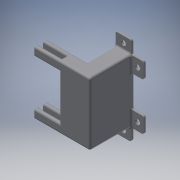
# Autodesk Inventor part: Tail_Base
Saved by Autodesk Inventor 2018 (Build 220112000, 112)
## iProperties
Created: 2017-11-24
Part Number: Tail_Base
Material: Generic
Document SubType Name: Modeling
Designer: reide
Density: 1 g/cm^3
Appearance: Default
Author: reide
Autodesk Inventor part; units mm, degrees
ref_plane "YZ Plane" through (0, 0, 0) normal (1, 0, 0) x (0, 1, 0)
ref_plane "XZ Plane" through (0, 0, 0) normal (0, 1, 0) x (-1, 0, 0)
ref_plane "XY Plane" through (0, 0, 0) normal (0, 0, 1) x (1, 0, 0)
sketch "Sketch1" plane through (0, 0, 0) normal (0, 0, 1) x (1, 0, 0)
  line L0 (0, -18.542) -> (0, -2.54) projected
  line L1 (0, -18.542) -> (-1.27, -18.542) projected
  line L2 (-11.43, -18.542) -> (-1.27, -18.542) projected
  line L3 (-11.43, -18.542) -> (-12.7, -18.542) projected
  line L4 (-12.7, -18.542) -> (-12.7, -2.54) projected
  line L5 (0, 0) -> (-12.7, 0) projected
  line L6 (-12.7, 0) -> (-12.7, -2.54) projected
  line L7 (0, -2.54) -> (-12.7, -2.54) projected
  line L8 (0, 0) -> (0, -2.54) projected
  line L9 (0, 0) -> (0, 4.318) projected
  line L10 (-6.35, 4.318) -> (-1.27, 4.318) projected
  line L11 (0, 4.318) -> (-1.27, 4.318) projected
  line L12 (-11.43, 4.318) -> (-6.35, 4.318) projected
  line L13 (-11.43, 4.318) -> (-12.7, 4.318) projected
  line L14 (-12.7, 0) -> (-12.7, 4.318) projected
  line L15 (-12.7, -2.54) -> (12.3, -2.54)
  line L16 (12.3, -2.54) -> (12.3, -4.54)
  line L17 (12.3, -4.54) -> (-12.7, -4.54)
  line L18 (-12.7, -4.54) -> (-12.7, -2.54)
  line L19 (-12.7, 0) -> (12.3, 0)
  line L20 (12.3, 0) -> (12.3, 2)
  line L21 (12.3, 2) -> (-12.7, 2)
  line L22 (-12.7, 2) -> (-12.7, 0)
  line L23 (0, -2.54) -> (12.3, -2.54)
  line L24 (12.3, -2.54) -> (12.3, 0)
  line L25 (12.3, 0) -> (0, 0)
  line L26 (528.25, 17.398) -> (-81.35, 17.398) projected
  line L27 (-12.7, 2) -> (7.6, 2)
  line L28 (7.6, -4.54) -> (15.6, -4.54)
  line L29 (15.6, -4.54) -> (15.6, 17.398)
  line L30 (15.6, 17.398) -> (7.6, 17.398)
  line L31 (7.6, 17.398) -> (7.6, -4.54)
  dimension "d0" = 25
  dimension "d1" = 2
  dimension "d2" = 2
  dimension "d3" = 20.3
  dimension "d4" = 8
  constraints: 32 end point, 7 parallel, 4 horizontal, 4 perpendicular, 3 point on line, 2 other
  measures "d0" distance of L16.end L17.end
  measures "d1" distance of L15.end L16.end
  measures "d2" distance of L19.end L20.end
  measures "d3" distance of L21.end L27.end
  measures "d4" distance between parallel lines of L31 L29
extrude "Extrusion1" add sketch "Sketch1" against normal blind 32.004 contours L17 L4 L7 L0 | L0 L15 L31 L17 | L31 L15 L16 L17 | L5 L14 L21 L9 | L9 L21 L31 L19 | L31 L19 L24 L15 | L16 L24 L20 L21 L31 L26 L29 L28 | L31 L21 L20 L19
sketch "Sketch2" plane through (-12.7, -4.54, 0) normal (0, -1, 0) x (1, 0, 0)
  line L0 (0, 0) -> (0, -32.004) projected
  line L1 (12.7, 0) -> (0, 0)
  line L2 (0, 0) -> (0, -32.004)
  line L3 (0, -32.004) -> (12.7, -32.004)
  line L4 (12.7, -32.004) -> (12.7, 0)
  line L5 (1.27, -4.572) -> (11.43, -4.572) projected
  line L6 (11.43, -27.432) -> (1.27, -27.432) projected
  line L7 (12.7, -27.432) -> (0, -27.432)
  line L8 (0, -27.432) -> (0, -4.572)
  line L9 (0, -4.572) -> (12.7, -4.572)
  line L10 (12.7, -4.572) -> (12.7, -27.432)
  constraints: 16 end point, 4 parallel, 2 horizontal, 2 perpendicular, 2 point on line
extrude "Extrusion2" cut sketch "Sketch2" against normal blind 32.004 contours L9 L5 L4 L7 L6 L0
sketch "Sketch3" plane through (7.6, 17.398, 0) normal (0, 1, 0) x (1, 0, 0)
  circle A0 centre (32.1372, -17.653) radius 1.5 projected
  circle A1 centre (80.358, -17.653) radius 1.5 projected
  circle A2 centre (83.533, 29.972) radius 1.5 projected
  circle A3 centre (32.1372, 39.497) radius 1.5 projected
  circle A4 centre (80.358, 39.497) radius 1.5 projected
  circle A5 centre (28.9622, 29.972) radius 1.5 projected
  circle A6 centre (56.2418, 39.497) radius 1.5 projected
  circle A7 centre (83.533, -8.128) radius 1.5 projected
  circle A8 centre (56.2534, -17.653) radius 1.5 projected
  circle A9 centre (28.9622, -8.128) radius 1.5 projected
  line L0 (86.708, -1.778) -> (25.7872, -1.778) projected
  line L1 (25.7872, -1.778) -> (25.7872, 23.622) projected
  line L2 (25.7872, 23.622) -> (86.708, 23.622) projected
  line L3 (86.708, 23.622) -> (86.708, -1.778) projected
  line L4 (290.8689, 60.2679) -> (290.8689, 56.2679) projected
  arc A10 (287.8691, 56.2679) -> (290.8689, 56.2679) centre (289.369, 56.2679) ccw projected
  line L5 (287.8691, 56.2679) -> (287.8691, 60.2679) projected
  arc A11 (290.8689, 60.2679) -> (287.8691, 60.2679) centre (289.369, 60.2679) ccw projected
  line L6 (226.1857, 60.2219) -> (226.1857, 56.2219) projected
  arc A12 (223.1859, 56.2219) -> (226.1857, 56.2219) centre (224.6858, 56.2219) ccw projected
  line L7 (223.1859, 56.2219) -> (223.1859, 60.2219) projected
  arc A13 (226.1857, 60.2219) -> (223.1859, 60.2219) centre (224.6858, 60.2219) ccw projected
  line L8 (290.9502, -54.235) -> (290.9502, -58.235) projected
  arc A14 (287.9504, -58.235) -> (290.9502, -58.235) centre (289.4503, -58.235) ccw projected
  line L9 (287.9504, -58.235) -> (287.9504, -54.235) projected
  arc A15 (290.9502, -54.235) -> (287.9504, -54.235) centre (289.4503, -54.235) ccw projected
  line L10 (226.1857, -54.281) -> (226.1857, -58.281) projected
  arc A16 (223.1859, -58.281) -> (226.1857, -58.281) centre (224.6858, -58.281) ccw projected
  line L11 (223.1859, -58.281) -> (223.1859, -54.281) projected
  arc A17 (226.1857, -54.281) -> (223.1859, -54.281) centre (224.6858, -54.281) ccw projected
  arc A18 (206.1145, 27.7587) -> (206.1146, 30.7563) centre (206.1145, 29.2575) ccw projected
  line L12 (206.1145, 27.7587) -> (202.1146, 27.7586) projected
  arc A19 (202.1146, 30.7565) -> (202.1146, 27.7586) centre (202.1145, 29.2575) ccw projected
  line L13 (202.1146, 30.7565) -> (206.1146, 30.7563) projected
  arc A20 (198.5105, -37.0167) -> (198.5105, -34.0191) centre (198.5105, -35.5179) ccw projected
  line L14 (198.5105, -37.0167) -> (194.5105, -37.0169) projected
  arc A21 (194.5106, -34.0189) -> (194.5105, -37.0169) centre (194.5105, -35.5179) ccw projected
  line L15 (194.5106, -34.0189) -> (198.5105, -34.0191) projected
  arc A22 (312.8978, 27.8346) -> (312.8979, 30.8322) centre (312.8978, 29.3334) ccw projected
  line L16 (312.8978, 27.8346) -> (308.8978, 27.8344) projected
  arc A23 (308.8979, 30.8324) -> (308.8978, 27.8344) centre (308.8978, 29.3334) ccw projected
  line L17 (308.8979, 30.8324) -> (312.8979, 30.8322) projected
  arc A24 (320.5507, -37.0114) -> (320.5509, -34.0138) centre (320.5507, -35.5126) ccw projected
  line L18 (320.5507, -37.0114) -> (316.5508, -37.0116) projected
  arc A25 (316.5508, -34.0136) -> (316.5508, -37.0116) centre (316.5507, -35.5126) ccw projected
  line L19 (316.5508, -34.0136) -> (320.5509, -34.0138) projected
  line L20 (312.9007, -37.0114) -> (308.9008, -37.0116) projected
  arc A26 (308.9008, -34.0136) -> (308.9008, -37.0116) centre (308.9008, -35.5126) ccw projected
  line L21 (308.9008, -34.0136) -> (312.9008, -34.0138) projected
  arc A27 (312.9007, -37.0114) -> (312.9008, -34.0138) centre (312.9008, -35.5126) ccw projected
  arc A28 (320.5047, 27.84) -> (320.5049, 30.8376) centre (320.5047, 29.3388) ccw projected
  line L22 (320.5047, 27.84) -> (316.5048, 27.8398) projected
  arc A29 (316.5048, 30.8378) -> (316.5048, 27.8398) centre (316.5047, 29.3388) ccw projected
  line L23 (316.5048, 30.8378) -> (320.5049, 30.8376) projected
  arc A30 (206.1605, -37.0163) -> (206.1606, -34.0187) centre (206.1605, -35.5175) ccw projected
  line L24 (206.1605, -37.0163) -> (202.1606, -37.0165) projected
  arc A31 (202.1606, -34.0185) -> (202.1606, -37.0165) centre (202.1605, -35.5175) ccw projected
  line L25 (202.1606, -34.0185) -> (206.1606, -34.0187) projected
  arc A32 (198.4646, 27.7533) -> (198.4645, 30.7509) centre (198.4645, 29.2521) ccw projected
  line L26 (198.4646, 27.7533) -> (194.4645, 27.7531) projected
  arc A33 (194.4646, 30.7511) -> (194.4645, 27.7531) centre (194.4645, 29.2521) ccw projected
  line L27 (194.4646, 30.7511) -> (198.4645, 30.7509) projected
  line L28 (223.1855, -65.931) -> (223.1855, -61.931) projected
  arc A34 (226.1854, -61.931) -> (223.1855, -61.931) centre (224.6854, -61.931) ccw projected
  line L29 (226.1854, -61.931) -> (226.1854, -65.931) projected
  arc A35 (223.1855, -65.931) -> (226.1854, -65.931) centre (224.6854, -65.931) ccw projected
  line L30 (290.9557, -61.931) -> (290.9557, -65.931) projected
  arc A36 (287.9558, -65.931) -> (290.9557, -65.931) centre (289.4558, -65.931) ccw projected
  line L31 (287.9558, -65.931) -> (287.9558, -61.931) projected
  arc A37 (290.9557, -61.931) -> (287.9558, -61.931) centre (289.4558, -61.931) ccw projected
  line L32 (226.1857, 52.5719) -> (226.1857, 48.5719) projected
  arc A38 (223.1859, 48.5719) -> (226.1857, 48.5719) centre (224.6858, 48.5719) ccw projected
  line L33 (223.1859, 48.5719) -> (223.1859, 52.5719) projected
  arc A39 (226.1857, 52.5719) -> (223.1859, 52.5719) centre (224.6858, 52.5719) ccw projected
  line L34 (290.8743, 52.6179) -> (290.8743, 48.6179) projected
  arc A40 (287.8745, 48.6179) -> (290.8743, 48.6179) centre (289.3744, 48.6179) ccw projected
  line L35 (287.8745, 48.6179) -> (287.8745, 52.6179) projected
  arc A41 (290.8743, 52.6179) -> (287.8745, 52.6179) centre (289.3744, 52.6179) ccw projected
  ellipse E0 centre (215.85, 10.922) end of major axis (-88.95, 10.922) minor radius 228.6 projected
  line L36 (8, 0) -> (0, 0) projected
  line L37 (8, 0) -> (8, 32.004) projected
  line L38 (0, 32.004) -> (8, 32.004) projected
  line L39 (8, 0) -> (0, 0)
  line L40 (0, 0) -> (0, -6.35)
  line L41 (0, -6.35) -> (8, -6.35)
  line L42 (8, -6.35) -> (8, 0)
  line L43 (8, 32.004) -> (-20.3, 32.004) projected
  line L44 (8, 32.004) -> (0, 32.004)
  line L45 (0, 32.004) -> (0, 38.354)
  line L46 (0, 38.354) -> (8, 38.354)
  line L47 (8, 38.354) -> (8, 32.004)
  circle A42 centre (4, 35.179) radius 1.5 projected
  circle A43 centre (4, -3.175) radius 1.5 projected
  line L48 (8, 32.004) -> (14.35, 32.004)
  line L49 (14.35, 32.004) -> (14.35, 24.004)
  line L50 (14.35, 24.004) -> (8, 24.004)
  line L51 (8, 0) -> (14.35, 0)
  line L52 (14.35, 0) -> (14.35, 8)
  line L53 (14.35, 8) -> (8, 8)
  circle A44 centre (4, 35.179) radius 1.25
  circle A45 centre (4, -3.175) radius 1.25
  circle A46 centre (11.175, 4) radius 1.25
  circle A47 centre (11.175, 28.004) radius 1.25
  point P0 (-7.6, 0)
  dimension "d9" = 6.35
  dimension "d10" = 6.35
  dimension "d21" = 6.35
  dimension "d22" = 8
  dimension "d23" = 8
  dimension "d24" = 2.5
  dimension "d25" = 2.5
  dimension "d26" = 2.5
  dimension "d27" = 2.5
  constraints: 28 end point, 5 point on line, 4 centre point, 4 parallel, 4 perpendicular, 3 horizontal, 2 coincident, 1 vertical, 1 other
  measures "d9" distance of L39.end L40.end
  measures "d10" distance of L44.end L45.end
  measures "d21" distance of L37.end L48.end
  measures "d22" distance of L48.end L49.end
  measures "d23" distance of L51.end L52.end
  measures "d24" diameter of A44
  measures "d25" diameter of A45
  measures "d26" diameter of A46
  measures "d27" diameter of A47
extrude "Extrusion3" add sketch "Sketch3" against normal blind 1 contours L42 L41 L40 L36 | L37 L53 L52 L51 | L38 L45 L46 L47 | L37 L48 L49 L50 | A42 | A43 | A44 | A45
sketch "Sketch4" plane through (7.6, 16.398, 0) normal (0, -1, 0) x (1, 0, 0)
  line L0 (8, 6.35) -> (0, 6.35) projected
  line L1 (0, -38.354) -> (8, -38.354) projected
  line L2 (0, -38.354) -> (0, 6.35) projected
  line L3 (0, -38.354) -> (0, -32.004)
  line L4 (8, -32.004) -> (-20.3, -32.004) projected
  line L5 (-20.3, 0) -> (8, 0) projected
  line L6 (0, 0) -> (0, 6.35)
  circle A0 centre (4, 3.175) radius 1.25
  circle A1 centre (4, -35.179) radius 1.25
  point P0 (-7.6, 0)
  point P1 (4, 6.35)
  point P2 (4, -38.354)
  point P3 (0, -35.179)
  point P4 (0, 3.175)
  dimension "d13" = 2.5
  dimension "d14" = 2.5
  constraints: 4 end point, 4 midpoint, 3 point on line, 2 centre point, 1 perpendicular, 1 vertical
  measures "d13" diameter of A0
  measures "d14" diameter of A1
extrude "Extrusion4" cut sketch "Sketch4" against normal blind 1
sketch "Sketch5" plane through (0, 0, 0) normal (0, 0, 1) x (1, 0, 0)
  line L0 (0, 0) -> (0, -2.54) projected
  line L1 (7.6, -2.54) -> (-12.7, -2.54) projected
  line L2 (-12.7, 0) -> (7.6, 0) projected
  line L3 (7.6, 0) -> (7.6, -2.54) projected
extrude "Extrusion5" add sketch "Sketch5" against normal blind 32.004
fillet "Fillet1" radius 1 18 edges at (11.6, 16.398, 0) (7.6, 16.898, 6.35) (15.6, 16.898, 6.35) (11.6, 16.398, -32.004) (7.6, 16.898, -38.354) (15.6, 16.898, -38.354) (15.6, 5.929, -32.004) (7.6, 9.199, -32.004) (7.6, 9.199, 0) (15.6, 5.929, 0) (15.6, 16.398, -28.004) (15.6, 16.398, -4) (21.95, 16.898, 0) (21.95, 16.898, -8) (21.95, 16.898, -24.004) (21.95, 16.898, -32.004) (15.6, 16.898, -24.004) (15.6, 16.898, -8)
fillet "Fillet2" radius 1 21 edges at (15.3071, -4.54, -0.2929) (15.6, -4.54, -16.002) (15.3071, -4.54, -31.7111) (0.95, -4.54, -32.004) (0.95, -4.54, 0) (-2.05, 2, -32.004) (0, 2, -16.002) (-6.35, 2, -4.572) (-2.05, 2, 0) (-6.35, 2, -27.432) (-6.35, -2.54, 0) (-6.35, -2.54, -4.572) (-6.35, -4.54, -4.572) (-6.35, 0, -4.572) (-6.35, 0, 0) (0, -4.54, -16.002) (-6.35, -4.54, -27.432) (-6.35, -2.54, -27.432) (-6.35, -2.54, -32.004) (-6.35, 0, -27.432) (-6.35, 0, -32.004)
body "Solid1"
